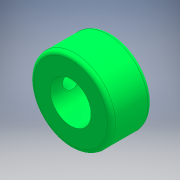
# Autodesk Inventor part: Anello d'arresto
Saved by Autodesk Inventor 2016 (Build 200138000, 138)
## iProperties
Created: 2016-09-10
Part Number: Anello d'arresto
Material: Generic
Document SubType Name: Modeling
Designer: Muhammad
Density: 1 g/cm^3
Appearance: Default
Author: Muhammad
Autodesk Inventor part; units mm, degrees
ref_plane "YZ Plane" through (0, 0, 0) normal (1, 0, 0) x (0, 1, 0)
ref_plane "XZ Plane" through (0, 0, 0) normal (0, 1, 0) x (-1, 0, 0)
ref_plane "XY Plane" through (0, 0, 0) normal (0, 0, 1) x (1, 0, 0)
sketch "Sketch1" plane through (0, 0, 0) normal (0, 1, 0) x (-1, 0, 0)
  circle A0 centre (0, 0) radius 2.5
  circle A1 centre (0, 0) radius 5
  constraints: 2 centre point, 2 coincident
extrude "Extrusion1" add sketch "Sketch1" along normal blind 5
fillet "Fillet1" radius 0.5 2 edges at (5, 5, 0) (5, 0, 0)
sketch "Sketch2" plane through (0, 0, 0) normal (1, 0, 0) x (0, 1, 0)
  line L0 (0, 0) -> (5, 0) construction
  line L1 (5, 2.5) -> (5, -2.5) construction
  circle A0 centre (2.5, 0) radius 1.5
  dimension "d5" = 3
  constraints: 2 end point, 2 midpoint, 1 centre point
  measures "d5" diameter of A0
extrude "Extrusion2" add sketch "Sketch2" against normal blind 5.25
sketch "Sketch3" plane through (-5.25, 2.5, 0) normal (-1, 0, 0) x (0, 0, 1)
  circle A0 centre (0, 0) radius 1
  point P0 (0, -2.5)
  dimension "d9" = 2
  constraints: 1 centre point
  measures "d9" diameter of A0
extrude "Extrusion3" cut sketch "Sketch3" against normal blind 5.25
sketch "Sketch4" plane through (0, 0, 0) normal (0, 1, 0) x (-1, 0, 0)
  circle A0 centre (0, 0) radius 2.5
  constraints: 1 centre point, 1 coincident
extrude "Extrusion4" cut sketch "Sketch4" along normal blind 5.25
fillet "Fillet2" radius 0.5 1 edges at (-5.25, 1, 0)
body "Solid1"
